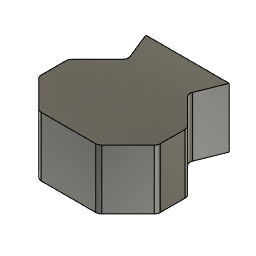
vase v2 (Autodesk Fusion 360 design; units mm, degrees)
Autodesk Fusion 360 part; units mm, degrees
note: some values were not read from the file. Chosen so that the rebuilt part matches the saved one: that a step has no effect. Set by a fixed rule: which sketch regions a step uses.
sketch "vase-side" plane through (0, 0, 0) normal (0, 0, 1) x (1, 0, 0)
  line L0 (0, 0) -> (45.8579, 0)
  line L1 (52.9289, 2.9289) -> (97.0711, 47.0711)
  line L2 (100, 54.1421) -> (100, 95.8579)
  line L3 (97.0711, 102.9289) -> (54.6626, 145.3374)
  line L4 (52.4489, 156.1223) -> (70, 200)
  line L5 (70, 200) -> (0, 200)
  line L6 (0, 200) -> (0, 0)
  line L7 (0, 0) -> (-45.8579, 0)
  line L8 (-52.9289, 2.9289) -> (-97.0711, 47.0711)
  line L9 (-100, 54.1421) -> (-100, 95.8579)
  line L10 (-97.0711, 102.9289) -> (-54.6626, 145.3374)
  line L11 (-52.4489, 156.1223) -> (-70, 200)
  line L12 (-70, 200) -> (0, 200)
  arc A0 (-54.6626, 145.3374) -> (-52.4489, 156.1223) centre (-61.7337, 152.4084) ccw
  arc A1 (52.4489, 156.1223) -> (54.6626, 145.3374) centre (61.7337, 152.4084) ccw
  arc A2 (-97.0711, 102.9289) -> (-100, 95.8579) centre (-90, 95.8579) ccw
  arc A3 (-100, 54.1421) -> (-97.0711, 47.0711) centre (-90, 54.1421) ccw
  arc A4 (-52.9289, 2.9289) -> (-45.8579, 0) centre (-45.8579, 10) ccw
  arc A5 (45.8579, 0) -> (52.9289, 2.9289) centre (45.8579, 10) ccw
  arc A6 (97.0711, 47.0711) -> (100, 54.1421) centre (90, 54.1421) ccw
  arc A7 (100, 95.8579) -> (97.0711, 102.9289) centre (90, 95.8579) ccw
  dimension "d8" = 10
  constraint coincident L0.start L6.end
  constraint horizontal L0
  constraint perpendicular L0 L2
  constraint perpendicular L1 L3
  constraint perpendicular L2 L5
  constraint perpendicular L0 L6
  constraint symmetric L0.start L6 L7.start
  constraint symmetric L4.end L6 L11.end
  constraint symmetric L5.end L6 L12.end
  constraint tangent L10 A0
  constraint tangent L11 A0
  constraint tangent L3 A1
  constraint tangent L4 A1
  constraint equal A0 A1
  constraint tangent L9 A2
  constraint tangent L10 A2
  constraint equal A0 A2
  constraint tangent L8 A3
  constraint tangent L9 A3
  constraint equal A0 A3
  constraint tangent L7 A4
  constraint tangent L8 A4
  constraint equal A0 A4
  constraint tangent L0 A5
  constraint tangent L1 A5
  constraint equal A0 A5
  constraint tangent L1 A6
  constraint tangent L2 A6
  constraint equal A0 A6
  constraint tangent L2 A7
  constraint tangent L3 A7
  constraint equal A0 A7
  measures "d8" radius of A0
extrude "Extrude1" add sketch "vase-side" along normal blind 100
fillet "Fillet1" [no effect]
fillet "Fillet2" [no effect]
fillet "Fillet3" [no effect]
cylinder "CylinderPrimitive1" cut diameter 72.111 height -180 placed x (1, 0, 0) y (0, 0, -1) z (0, 1, 0) at (0, 200, 50)
named bodies: "vase"
